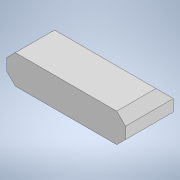
# Autodesk Inventor part: Magazin_Stössel
Saved by Autodesk Inventor 2021 (Build 250183000, 183)
## iProperties
Created: 2024-05-14
Part Number: Magazin_Stössel
Material: Generic
Document SubType Name: Modeling
Designer: Lukas
Density: 1 g/cm^3
Appearance: Default
Author: Lukas
Autodesk Inventor part; units mm, degrees
ref_plane "YZ Plane" through (0, 0, 0) normal (1, 0, 0) x (0, 1, 0)
ref_plane "XZ Plane" through (0, 0, 0) normal (0, 1, 0) x (-1, 0, 0)
ref_plane "XY Plane" through (0, 0, 0) normal (0, 0, 1) x (1, 0, 0)
sketch "Sketch1" plane through (0, 0, 0) normal (0, 0, 1) x (1, 0, 0)
  line L0 (-20, 2) -> (-17, 5)
  line L1 (-17, 5) -> (17, 5)
  line L2 (17, 5) -> (20, 2)
  line L3 (20, 2) -> (20, -2)
  line L4 (20, -2) -> (17, -5)
  line L5 (17, -5) -> (-17, -5)
  line L6 (-17, -5) -> (-20, -2)
  line L7 (-20, -2) -> (-20, 2)
  line L8 (16.9379, 4.85) -> (-16.9379, 4.85)
  line L9 (-16.9379, 4.85) -> (-19.85, 1.9379)
  line L10 (-19.85, 1.9379) -> (-19.85, -1.9379)
  line L11 (-19.85, -1.9379) -> (-16.9379, -4.85)
  line L12 (-16.9379, -4.85) -> (16.9379, -4.85)
  line L13 (16.9379, -4.85) -> (19.85, -1.9379)
  line L14 (19.85, -1.9379) -> (19.85, 1.9379)
  line L15 (19.85, 1.9379) -> (16.9379, 4.85)
  point P0 (0, 0)
  point P1 (0, 5)
  point P2 (-20, 0)
  dimension "d0" = 3
  dimension "d1" = 3
  dimension "d2" = 10
  dimension "d3" = 34
  dimension "d4" = 0.15
  constraints: 32 end point, 9 perpendicular, 4 parallel, 2 midpoint, 2 vertical alignment, 1 horizontal, 1 horizontal alignment, 7 other
  measures "d0" horizontal distance of L0.start L0.end
  measures "d1" horizontal distance of L0.start L0.end
  measures "d2" distance between parallel lines of L5 L1
  measures "d3" distance of L0.end L1.end
  measures "d4" distance between parallel lines of L1 L8
extrude "Extrusion1" add sketch "Sketch1" along normal blind 16 contours L15 L14 L13 L12 L11 L10 L9 L8
chamfer "Chamfer1" distance 2.9 angle 45 2 edges at (0, -4.85, 0) (0, 4.85, 0)
sketch "Sketch4" plane through (-16.9379, -4.85, 16) normal (0, -1, 0) x (1, 0, 0)
  line L0 (24.9379, -7) -> (8.9379, -7)
  line L1 (8.9379, -7) -> (8.9379, -11)
  line L2 (8.9379, -11) -> (24.9379, -11)
  line L3 (24.9379, -11) -> (24.9379, -7)
  line L4 (0, 0) -> (33.8757, 0) projected
  point P0 (16.9379, -16)
  point P1 (16.9379, 0)
  point P2 (16.9379, -7)
  dimension "d24" = 7
  dimension "d25" = 4
  dimension "d26" = 16
  constraints: 8 end point, 2 midpoint, 2 parallel, 1 horizontal, 1 perpendicular, 1 vertical alignment
  measures "d24" distance between parallel lines of L4 L0
  measures "d25" distance of L2.end L0.start
  measures "d26" distance of L1.end L2.end
extrude "Extrusion4" add sketch "Sketch4" along normal blind 3
chamfer "Chamfer2" distance 3 angle 45 2 edges at (-8, -4.85, 7) (8, -4.85, 7)
body "Solid1"
